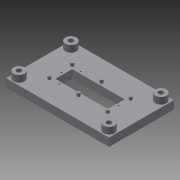
# Autodesk Inventor part: 490HV_MicrofluidicClamp
Saved by Autodesk Inventor 2015 (Build 190159000, 159)
## iProperties
Created: 2014-09-25
Part Number: 490HV_MicrofluidicClamp
Material: Generic
Document SubType Name: Modeling
Designer: Alex
Density: 1 g/cm^3
Appearance: Default
Author: Alex
Autodesk Inventor part; units mm, degrees
ref_plane "YZ Plane" through (0, 0, 0) normal (1, 0, 0) x (0, 1, 0)
ref_plane "XZ Plane" through (0, 0, 0) normal (0, 1, 0) x (-1, 0, 0)
ref_plane "XY Plane" through (0, 0, 0) normal (0, 0, 1) x (1, 0, 0)
sketch "Sketch1" plane through (0, 0, 0) normal (0, 1, 0) x (-1, 0, 0)
  line L0 (5.1091, 27.5) -> (-62.3909, 27.5)
  line L1 (-62.3909, 27.5) -> (-62.3909, -15)
  line L2 (-62.3909, -15) -> (5.1091, -15)
  line L3 (5.1091, -15) -> (5.1091, 27.5)
  line L4 (5.1091, 6.25) -> (-62.3909, 6.25)
  point P0 (0, 0)
  dimension "d0" = 42.5
  dimension "d1" = 67.5
  constraints: 10 end point, 2 midpoint, 2 parallel, 2 perpendicular, 1 horizontal, 1 other
  measures "d0" distance of L2.end L0.start
  measures "d1" distance of L1.end L2.end
extrude "Extrusion1" add sketch "Sketch1" along normal blind 5.31
sketch "Sketch2" plane through (0, 5.31, 0) normal (0, 1, 0) x (1, 0, 0)
  circle A0 centre (9.9709, -6.25) radius 0.5
  circle A1 centre (15.6009, -13.28) radius 0.5
  circle A2 centre (15.6009, 0.78) radius 0.5
  circle A3 centre (47.3109, -6.25) radius 0.5
  line L0 (-5.1091, -6.25) -> (62.3909, -6.25) construction
  line L1 (15.6009, 15.6122) -> (15.6009, -24.3614) construction
  line L2 (11.4709, -11.78) -> (45.8109, -11.78)
  line L3 (45.8109, -11.78) -> (45.8109, -0.72)
  line L4 (45.8109, -0.72) -> (11.4709, -0.72)
  line L5 (11.4709, -0.72) -> (11.4709, -11.78)
  circle A4 centre (-0.8591, 10.75) radius 1.625
  line L6 (62.3909, 15) -> (-5.1091, 15)
  circle A5 centre (-0.8591, -23.25) radius 1.625
  line L7 (-5.1091, -27.5) -> (62.3909, -27.5)
  circle A6 centre (58.1409, 10.75) radius 1.625
  circle A7 centre (58.1409, -23.25) radius 1.625
  line L8 (62.3909, -27.3764) -> (62.3909, 12.6236)
  line L9 (28.6409, -27.5) -> (28.6409, 15) construction
  line L10 (62.3909, -27.5) -> (62.3909, 15) projected
  line L11 (-5.1091, -27.5) -> (62.3909, -27.5) projected
  line L12 (-5.1091, 15) -> (-5.1091, -27.5) projected
  line L13 (62.3909, 15) -> (-5.1091, 15) projected
  point P0 (0, 0)
  dimension "d4" = 1
  dimension "d15" = 14.06
  dimension "d23" = 37.34
  dimension "d39" = 5.63
  dimension "d70" = 4.25
  dimension "d79" = 3.25
  dimension "d82" = 1
  dimension "d83" = 1
  dimension "d84" = 1
  dimension "d85" = 1
  dimension "d90" = 4.25
  dimension "d91" = 4.25
  dimension "d93" = 34
  dimension "d94" = 59
  dimension "d100" = 11.06
  constraints: 20 end point, 8 centre point, 6 equal radius, 6 point on line, 4 midpoint, 4 symmetric about line, 3 collinear, 2 parallel, 1 horizontal, 1 perpendicular, 1 vertical, 2 other
  measures "d4" diameter of A0
  measures "d15" distance of A2.centre A1.centre
  measures "d23" distance of A0.centre A3.centre
  measures "d39" horizontal distance of A1.centre A0.centre
  measures "d70" distance from line of A4.centre L6
  measures "d79" diameter of A5
  measures "d82" distance edge to line of A0 L5
  measures "d83" distance edge to line of A3 L3
  measures "d84" distance edge to line of A1 L2
  measures "d85" distance edge to line of A2 L4
  measures "d90" distance from line of L12 A4.centre
  measures "d91" distance from line of L10 A7.centre
  measures "d93" distance of A6.centre A7.centre
  measures "d94" distance of A7.centre A5.centre
  measures "d100" distance of L2.end L4.start
extrude "Extrusion2" cut sketch "Sketch2" against normal through all contours A0 | A1 | A2 | A3 | L5 L4 L3 L2 | A4 | A5 | A6 | A7
sketch "Sketch4" plane through (0, 5.31, 0) normal (0, 1, 0) x (1, 0, 0)
  circle A0 centre (-0.8591, 10.75) radius 3.625
  circle A1 centre (58.1409, -23.25) radius 3.625
  circle A2 centre (58.1409, 10.75) radius 3.625
  circle A3 centre (-0.8591, -23.25) radius 3.625
  circle A4 centre (-0.8591, -23.25) radius 1.625 construction
  circle A5 centre (58.1409, -23.25) radius 1.625 construction
  circle A6 centre (-0.8591, 10.75) radius 1.625 construction
  circle A7 centre (58.1409, 10.75) radius 1.625 construction
  circle A8 centre (58.1409, -23.25) radius 1.625
  circle A9 centre (-0.8591, -23.25) radius 1.625
  circle A10 centre (-0.8591, 10.75) radius 1.625
  circle A11 centre (58.1409, 10.75) radius 1.625
  circle A12 centre (47.8109, -13.78) radius 1
  circle A13 centre (9.4709, -13.78) radius 1
  circle A14 centre (47.8109, 1.28) radius 1
  circle A15 centre (9.4709, 1.28) radius 1
  line L0 (45.8109, -11.78) -> (11.4709, -11.78) projected
  line L1 (45.8109, -0.72) -> (45.8109, -11.78) projected
  line L2 (28.6409, -33.9575) -> (28.6409, 25.5773) construction
  line L3 (71.7292, -6.25) -> (-26.8251, -6.25) construction
  line L4 (47.8109, -13.78) -> (9.4709, -13.78) construction
  line L5 (47.8109, 1.28) -> (9.4709, 1.28) construction
  circle A16 centre (28.6409, 1.28) radius 1
  circle A17 centre (28.6409, -13.78) radius 1
  point P0 (0, 0)
  point P1 (56.8909, 12)
  point P2 (-2.1091, 12)
  dimension "d92" = 2
  dimension "d95" = 2
  dimension "d96" = 2
  dimension "d97" = 2
  constraints: 14 centre point, 12 equal radius, 8 end point, 5 symmetric about line, 4 coincident, 4 concentric, 2 midpoint, 2 point on line, 1 horizontal, 1 parallel
  measures "d92" radial gap between concentric circles of A0 A6
  measures "d95" diameter of A12
  measures "d96" distance from line of L4.start L0
  measures "d97" distance from line of L4.start L1
extrude "Extrusion4" add sketch "Sketch4" along normal blind 2
sketch "Sketch5" plane through (58.1409, 7.31, -10.75) normal (0, 1, 0) x (1, 0, 0)
  circle A0 centre (0, -34) radius 1.625 projected
  circle A1 centre (0, -34) radius 1
  circle A2 centre (0, -34) radius 3.625
  circle A3 centre (-59, -34) radius 1.625 projected
  circle A4 centre (-59, -34) radius 1.625
  circle A5 centre (-59, -34) radius 3.625
  circle A6 centre (-59, -34) radius 1.625 projected
  circle A7 centre (-59, -34) radius 3.625 projected
  circle A8 centre (0, -34) radius 3.625 projected
  circle A9 centre (-59, 0) radius 1.625
  circle A10 centre (0, 0) radius 1.625
  circle A11 centre (-59, 0) radius 3.625
  circle A12 centre (0, 0) radius 3.625
  circle A13 centre (0, 0) radius 3.625 projected
  circle A14 centre (0, 0) radius 1.625 projected
  circle A15 centre (-59, 0) radius 1.625 projected
  circle A16 centre (-59, 0) radius 3.625 projected
  point P0 (-58.1409, -10.75)
  constraints: 11 concentric, 8 centre point, 4 coincident
extrude "Extrusion5" add sketch "Sketch5" along normal blind 2.3 contours A2 | A5 | A11 | A12
equation "\"d31\" = d69"
equation "\"d69\" = 3"
body "Solid1"
